608zz (Autodesk Fusion 360 design; units mm, degrees)
Autodesk Fusion 360 part; units mm, degrees
sketch "Sketch1" plane through (0, 0, 0) normal (0, 1, 0) x (1, 0, 0)
  circle A0 centre (0, 0) radius 4
  circle A1 centre (0, 0) radius 11
  dimension "d1" = 8
  dimension "d2" = 22
  constraint coincident A0.centre A1.centre
  measures "d1" diameter of A0
  measures "d2" diameter of A1
extrude "Extrude1" add sketch "Sketch1" along normal blind 7
sketch "Sketch2" plane through (0, 0, 0) normal (0, -1, 0) x (1, 0, 0)
  circle A0 centre (0, 0) radius 4
  circle A1 centre (0, 0) radius 11
  circle A2 centre (0, 0) radius 10
  circle A3 centre (0, 0) radius 5
  dimension "d5" = 1
  dimension "d6" = 1
  constraint concentric A0 A2
  constraint concentric A0 A3
  measures "d5" distance of A0 A3
  measures "d6" distance of A1 A2
sketch "Sketch3" plane through (0, 7, 0) normal (0, 1, 0) x (-1, 0, 0)
  circle A0 centre (0, 0) radius 4
  circle A1 centre (0, 0) radius 11
  circle A2 centre (0, 0) radius 5
  circle A3 centre (0, 0) radius 10
  dimension "d7" = 1
  dimension "d8" = 1
  constraint concentric A0 A2
  constraint concentric A2 A3
  measures "d7" distance of A1 A3
  measures "d8" distance of A0 A2
extrude "Extrude2" cut sketch "Sketch3" against normal blind 0.01 contours A3
extrude "Extrude3" cut sketch "Sketch2" against normal blind 0.01 contours A2
equation "d6 = d5"
equation "d8 = d7"
